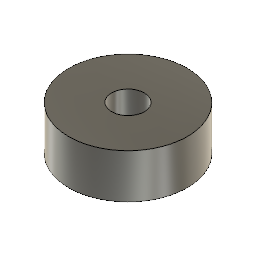
4mm_Wheel_Plug (Autodesk Fusion 360 design; units mm, degrees)
Autodesk Fusion 360 part; units mm, degrees
sketch "Sketch1" plane through (0, 0, 0) normal (0, 0, 1) x (1, 0, 0)
  circle A0 centre (0.6, 0.9) radius 2
  dimension "d1" = 4
  measures "d1" diameter of A0
extrude "Extrude1" add sketch "Sketch1" along normal blind 1.5
sketch "Sketch2" plane through (0, 0, 1.5) normal (0, 0, 1) x (-1, 0, 0)
  circle A0 centre (-0.6, -0.9) radius 2
  circle A1 centre (-0.6, -0.9) radius 0.55
  dimension "d4" = 1.1
  constraint concentric A0 A1
  measures "d4" diameter of A1
extrude "Extrude2" cut sketch "Sketch2" against normal blind 3.1 contours A1
